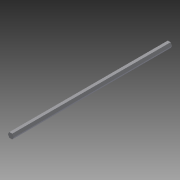
# Autodesk Inventor part: bigShaft
Saved by Autodesk Inventor 2014 SP2 (Build 180246200, 246)
## iProperties
Created: 2016-04-21
Part Number: bigShaft
Material: Generic
Document SubType Name: Modeling
Designer: Administrator
Density: 1 g/cm^3
Appearance: Default
Author: Administrator
Autodesk Inventor part; units mm, degrees
ref_plane "YZ Plane" through (0, 0, 0) normal (1, 0, 0) x (0, 1, 0)
ref_plane "XZ Plane" through (0, 0, 0) normal (0, 1, 0) x (-1, 0, 0)
ref_plane "XY Plane" through (0, 0, 0) normal (0, 0, 1) x (1, 0, 0)
sketch "Sketch1" plane through (0, 0, 0) normal (0, 0, 1) x (1, 0, 0)
  line L0 (0, 6.35) -> (-3.6703, 6.35)
  line L1 (-3.6703, 6.35) -> (-7.3282, 0)
  line L2 (-7.3282, 0) -> (-3.6703, -6.35)
  line L3 (-3.6703, -6.35) -> (0, -6.35)
  line L4 (0, 6.35) -> (3.6703, 6.35)
  line L5 (3.6703, 6.35) -> (7.3282, 0)
  line L6 (7.3282, 0) -> (3.6703, -6.35)
  line L7 (3.6703, -6.35) -> (0, -6.35)
  point P0 (0, 0)
  dimension "d1" = 6.35
  dimension "d2" = 3.6703
  dimension "d4" = 3.6703
  dimension "d5" = 12.7
  dimension "d6" = 12.7
  dimension "d7" = 12.7
  constraints: 16 end point, 2 parallel
  measures "d1" distance of point (0, 0) L3.end
  measures "d2" distance of L0.start L0.end
  measures "d4" distance of L2.end L3.end
  measures "d5" distance between parallel lines of L6 L1
  measures "d6" distance between parallel lines of L2 L5
  measures "d7" distance of L3.end L0.start
extrude "Extrusion1" add sketch "Sketch1" along normal blind 406.4
body "Solid1"
